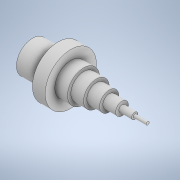
# Autodesk Inventor part: 零件3
Saved by Autodesk Inventor 2020 (Build 240168000, 168)
## iProperties
Created: 2020-12-28
Part Number: 零件3
Material: 一般
Document SubType Name: Modeling
Designer: User
Density: 1 g/cm^3
Appearance: 預設
Author: User
Autodesk Inventor part; units mm, degrees
ref_plane "YZ Plane" through (0, 0, 0) normal (1, 0, 0) x (0, 1, 0)
ref_plane "XZ Plane" through (0, 0, 0) normal (0, 1, 0) x (-1, 0, 0)
ref_plane "XY Plane" through (0, 0, 0) normal (0, 0, 1) x (1, 0, 0)
sketch "草圖1" plane through (0, 0, 0) normal (0, 0, 1) x (1, 0, 0)
  line L0 (0, 0) -> (0, 635)
  line L1 (0, 635) -> (1016, 635)
  line L2 (1016, 635) -> (1016, 1016)
  line L3 (1016, 1016) -> (1524, 1016)
  line L4 (1524, 1016) -> (1524, 635)
  line L5 (1524, 635) -> (2032, 635)
  line L6 (2032, 635) -> (2032, 508)
  line L7 (2032, 508) -> (2540, 508)
  line L8 (2540, 508) -> (2540, 381)
  line L9 (2540, 381) -> (3048, 381)
  line L10 (3048, 381) -> (3048, 254)
  line L11 (3048, 254) -> (3556, 254)
  line L12 (3556, 254) -> (3556, 127)
  line L13 (3556, 0) -> (0, 0)
  line L14 (3556, 254) -> (3556, 127)
  line L15 (3556, 127) -> (4064, 127)
  line L16 (4064, 127) -> (4064, 0)
  line L17 (4064, 0) -> (3556, 0)
  dimension "d0" = 635
  dimension "d1" = 1016
  dimension "d2" = 381
  dimension "d3" = 508
  dimension "d4" = 508
  dimension "d5" = 127
  dimension "d6" = 508
  dimension "d7" = 127
  dimension "d8" = 508
  dimension "d9" = 127
  dimension "d10" = 508
  dimension "d11" = 127
  dimension "d12" = 508
  constraints: 36 end point, 15 perpendicular, 2 point on line, 1 vertical
  measures "d0" distance of L0.start L0.end
  measures "d1" distance of L0.end L1.end
  measures "d2" distance of L1.end L2.end
  measures "d3" distance of L2.end L3.end
  measures "d4" distance of L4.end L5.end
  measures "d5" distance of L5.end L6.end
  measures "d6" distance of L6.end L7.end
  measures "d7" distance of L7.end L8.end
  measures "d8" distance of L8.end L9.end
  measures "d9" distance of L9.end L10.end
  measures "d10" distance of L10.end L11.end
  measures "d11" distance of L12.end L11.end
  measures "d12" distance of L12.end L15.end
revolve "迴轉1" add sketch "草圖1" angle 360 about axis through (3556, 0, 0) along (-1, 0, 0)
sketch "草圖2" plane through (0, 0, 0) normal (-1, 0, 0) x (0, 0, 1)
  circle A0 centre (0, 0) radius 127 projected
  circle A1 centre (0, 0) radius 508
  dimension "d14" = 1016
  constraints: 1 centre point, 1 coincident
  measures "d14" diameter of A1
extrude "擠出1" cut sketch "草圖2" against normal blind 1016 contours A0 | A1
sketch "草圖3" plane through (4064, 0, 0) normal (1, 0, 0) x (0, 0, -1)
  circle A0 centre (0, 0) radius 127 projected
  circle A1 centre (0, 0) radius 63.5
  dimension "d17" = 127
  constraints: 1 centre point, 1 coincident
  measures "d17" diameter of A1
extrude "擠出2" add sketch "草圖3" along normal blind 508 contours A1
